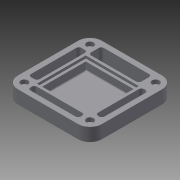
# Autodesk Inventor part: new IC holder2
Saved by Autodesk Inventor 2015 (Build 190159000, 159)
## iProperties
Created: 2014-12-11
Part Number: new IC holder2
Material: Generic
Document SubType Name: Modeling
Designer: Purple
Density: 1 g/cm^3
Appearance: Default
Author: Purple
Autodesk Inventor part; units mm, degrees
ref_plane "YZ Plane" through (0, 0, 0) normal (1, 0, 0) x (0, 1, 0)
ref_plane "XZ Plane" through (0, 0, 0) normal (0, 1, 0) x (-1, 0, 0)
sketch "Sketch1" plane through (0, 0, 0) normal (0, 1, 0) x (-1, 0, 0)
  line L0 (30, 30) -> (-30, 30)
  line L1 (-30, 30) -> (-30, -30)
  line L2 (-30, -30) -> (30, -30)
  line L3 (30, -30) -> (30, 30)
  line L4 (30, 30) -> (-30, -30) construction
  line L5 (-30, 30) -> (30, -30) construction
  point P0 (0, 0)
  dimension "d0" = 60
  dimension "d1" = 60
  constraints: 12 end point, 2 midpoint, 2 parallel, 1 horizontal, 1 perpendicular
  measures "d0" distance of L2.end L1.end
  measures "d1" distance of L0.end L1.end
extrude "Extrusion1" add sketch "Sketch1" along normal blind 10
fillet "Fillet1" radius 7 4 edges at (30, 5, 30) (30, 5, -30) (-30, 5, 30) (-30, 5, -30)
sketch "Sketch2" plane through (0, 10, 0) normal (0, 1, 0) x (1, 0, 0)
  line L0 (-30, 30) -> (30, 30)
  line L1 (30, 30) -> (30, -30)
  line L2 (30, -30) -> (-30, -30)
  line L3 (-30, -30) -> (-30, 30)
  line L4 (-30, 30) -> (30, -30) construction
  line L5 (30, 30) -> (-30, -30) construction
  line L6 (25, -25) -> (25, 25)
  line L7 (25, 25) -> (-25, 25)
  line L8 (-25, 25) -> (-25, -25)
  line L9 (-25, -25) -> (25, -25)
  circle A0 centre (25, -25) radius 2.75
  circle A1 centre (-25, -25) radius 2.75
  circle A2 centre (25, 25) radius 2.75
  circle A3 centre (-25, 25) radius 2.75
  point P0 (0, 0)
  dimension "d5" = 5
  dimension "d6" = 5.5
  dimension "d7" = 5.5
  dimension "d8" = 5.5
  dimension "d9" = 5.5
  constraints: 20 end point, 4 centre point, 4 coincident, 4 parallel, 2 midpoint, 2 perpendicular, 1 horizontal, 3 other
  measures "d5" distance between parallel lines of L1 L6
  measures "d6" diameter of A0
  measures "d7" diameter of A1
  measures "d8" diameter of A2
  measures "d9" diameter of A3
extrude "Extrusion2" cut sketch "Sketch2" against normal blind 3 contours L9 A0 L6 | L6 A0 L9 | A2 L7 L6 | L6 L7 A2 | A1 L8 L9 | L9 L8 A1 | A3 L8 L7 | L7 L8 A3
sketch "Sketch7" plane through (0, 10, 0) normal (0, 1, 0) x (1, 0, 0)
  line L0 (-23, 30) -> (23, 30)
  line L1 (30, 23) -> (30, -23)
  line L2 (23, -30) -> (-23, -30)
  line L3 (-30, -23) -> (-30, 23)
  line L4 (-30, 30) -> (30, -30) construction
  line L5 (30, 30) -> (-30, -30) construction
  arc A0 (-23, 30) -> (-30, 23) centre (-23, 23) ccw
  arc A1 (-30, -23) -> (-23, -30) centre (-23, -23) ccw
  arc A2 (23, -30) -> (30, -23) centre (23, -23) ccw
  arc A3 (30, 23) -> (23, 30) centre (23, 23) ccw
  line L6 (23, 32) -> (-23, 32)
  arc A4 (-23, 32) -> (-32, 23) centre (-23, 23) ccw
  line L7 (-32, 23) -> (-32, -23)
  arc A5 (-32, -23) -> (-23, -32) centre (-23, -23) ccw
  line L8 (-23, -32) -> (23, -32)
  arc A6 (23, -32) -> (32, -23) centre (23, -23) ccw
  line L9 (32, -23) -> (32, 23)
  arc A7 (32, 23) -> (23, 32) centre (23, 23) ccw
  point P0 (0, 0)
  dimension "d47" = 7
  dimension "d48" = 2
  constraints: 20 end point, 16 point on circle, 8 centre point, 8 point on line, 8 tangent, 4 parallel, 3 equal radius, 2 midpoint, 2 perpendicular, 1 horizontal, 7 other
  measures "d47" radius of A0
  measures "d48" distance between parallel lines of L0 L6
extrude "Extrusion6" add sketch "Sketch7" against normal blind 10
sketch "Sketch11" plane through (0, 10, 0) normal (0, 1, 0) x (1, 0, 0)
  circle A0 centre (25, -25) radius 2.75 projected
  line L0 (-25, 25) -> (25, 25)
  line L1 (25, 25) -> (25, -25)
  line L2 (25, -25) -> (-25, -25)
  line L3 (-25, -25) -> (-25, 25)
  line L4 (-25, 25) -> (25, -25) construction
  line L5 (25, 25) -> (-25, -25) construction
  line L6 (21, -21) -> (21, 16.2)
  line L7 (-19.4, -21) -> (21, -21)
  line L8 (-19.4, -21) -> (-19.4, 16.2)
  line L9 (21, 16.2) -> (-19.4, 16.2)
  line L10 (-17.4, 14.2) -> (-17.4, -19)
  line L11 (-17.4, -19) -> (19, -19)
  line L12 (19, -19) -> (19, 14.2)
  line L13 (19, 14.2) -> (-17.4, 14.2)
  point P0 (0, 0)
  dimension "d66" = 4
  dimension "d67" = 40.4
  dimension "d68" = 37.2
  dimension "d69" = 2
  constraints: 28 end point, 3 perpendicular, 2 midpoint, 2 parallel, 1 horizontal, 1 vertical, 3 other
  measures "d66" distance between parallel lines of L1 L6
  measures "d67" distance of L7.start L6.start
  measures "d68" distance of L6.end L6.start
  measures "d69" distance between parallel lines of L9 L13
extrude "Extrusion9" cut sketch "Sketch11" against normal blind 2 contours L7 L8 L9 L6
sketch "Sketch12" plane through (0, 10, 0) normal (0, 1, 0) x (1, 0, 0)
  line L0 (-17.4, 14.2) -> (19, 14.2)
  line L1 (19, 14.2) -> (19, -19)
  line L2 (19, -19) -> (-17.4, -19)
  line L3 (-17.4, -19) -> (-17.4, 14.2)
  point P0 (0, 0)
  constraints: 8 end point, 2 parallel, 1 horizontal, 1 perpendicular
extrude "Extrusion10" cut sketch "Sketch12" against normal blind 8
sketch "Sketch13" plane through (0, 10, 0) normal (0, 1, 0) x (1, 0, 0)
  line L0 (23, 32) -> (-23, 32) projected
  line L1 (-19.4, 18.2) -> (-19.4, 28)
  line L2 (-19.4, 28) -> (19, 28)
  line L3 (-19.4, 18.2) -> (19, 18.2)
  line L4 (32, -23) -> (32, 23) projected
  line L5 (21, 16.2) -> (21, -21) projected
  line L6 (28, 16.2) -> (23, 16.2)
  line L7 (23, 16.2) -> (23, -19)
  line L8 (28, -19) -> (28, 16.2)
  line L9 (23, -19) -> (28, -19)
  line L10 (21, -21) -> (-19.4, -21) projected
  line L11 (-23, -32) -> (23, -32) projected
  line L12 (19, -28) -> (19, -23)
  line L13 (19, -28) -> (-19.4, -28)
  line L14 (-19.4, -28) -> (-19.4, -23)
  line L15 (-19.4, -23) -> (19, -23)
  line L16 (19, 18.2) -> (19, 28)
  line L17 (19, 14.2) -> (19, -19) projected
  line L18 (-32, 23) -> (-32, -23) projected
  line L19 (-19.4, -21) -> (-19.4, 16.2) projected
  line L20 (-28, -19) -> (-28, 19.5)
  line L21 (-28, -19) -> (-21.4, -19)
  line L22 (-21.4, -19) -> (-21.4, 19.5)
  line L23 (-28, 19.5) -> (-21.4, 19.5)
  dimension "d77" = 2
  dimension "d78" = 4
  dimension "d81" = 2
  dimension "d84" = 2
  dimension "d87" = 4
  dimension "d88" = 4
  dimension "d89" = 2
  dimension "d90" = 38.5
  constraints: 32 end point, 4 horizontal, 4 perpendicular, 3 vertical, 1 collinear, 1 parallel
  measures "d77" distance of L1.start L19.end
  measures "d78" distance from line of L4 L6.start
  measures "d81" distance of L5.start L6.end
  measures "d84" distance from line of L10 L14.end
  measures "d87" distance from line of L11 L13.end
  measures "d88" distance from line of L20.start L18
  measures "d89" distance from line of L19 L21.end
  measures "d90" distance of L20.start L20.end
extrude "Extrusion11" cut sketch "Sketch13" against normal through all
fillet "Fillet3" radius 2 16 edges at (-19.4, 5, -28) (-28, 5, -19.5) (23, 5, -16.2) (-19.4, 5, 23) (19, 5, -28) (-21.4, 5, -19.5) (28, 5, -16.2) (19, 5, 23) (19, 5, -18.2) (28, 5, 19) (19, 5, 28) (-21.4, 5, 19) (-19.4, 5, -18.2) (23, 5, 19) (-19.4, 5, 28) (-28, 5, 19)
fillet "Fillet3" radius 1 4 edges at (0.8, 2, -14.2) (19, 2, 2.4) (-17.4, 2, 2.4) (0.8, 2, 19)
ref_plane "Work Plane2" through (0, 5, 0) normal (0, 1, 0) x (1, 0, 0)
mirror "Mirror2" about plane through (0, 5, 0) normal (0, 1, 0) of "Extrusion2"
body "Solid1"
